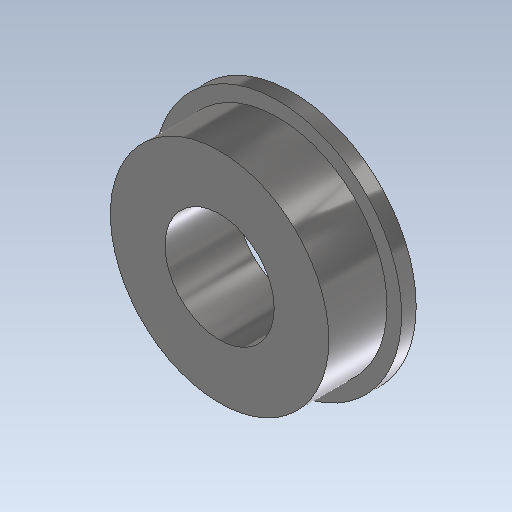
# Autodesk Inventor part: ベアリングHd6-D12-B4
Saved by Autodesk Inventor 2020.2 (Build 242310000, 310)
## iProperties
Created: 2017-02-12
Part Number: ベアリングHd6-D12-B4
Material: 鋼、炭素鋼
Document SubType Name: Modeling
Designer: 大空
Mass: 0.77 g
Surface Area: 4.64202 cm^2
Volume: 0.365028 cm^3
Density: 2.10943 g/cm^3
Appearance: 半つや出し
Author: 大空
Autodesk Inventor part; units mm, degrees
ref_plane "YZ Plane" through (0, 0, 0) normal (1, 0, 0) x (0, 1, 0)
ref_plane "XZ Plane" through (0, 0, 0) normal (0, 1, 0) x (-1, 0, 0)
ref_plane "XY Plane" through (0, 0, 0) normal (0, 0, 1) x (1, 0, 0)
sketch "スケッチ1" plane through (0, 0, 0) normal (0, 0, 1) x (1, 0, 0)
  circle A0 centre (0, 0) radius 3
  circle A1 centre (0, 0) radius 6
  circle A2 centre (0, 0) radius 6.8
  dimension "d0" = 6
  dimension "d1" = 12
  dimension "d13" = 0.8
  constraints: 3 centre point, 2 coincident
  measures "d0" diameter of A0
  measures "d1" diameter of A1
  measures "d13" radial gap between concentric circles of A1 A2
extrude "押し出し1" add sketch "スケッチ1" along normal blind 4 contours A1
extrude "押し出し5" add sketch "スケッチ1" along normal blind 0.8 contours A2
